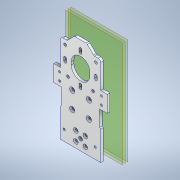
# Autodesk Inventor part: Printhead Base Plate REVI
Saved by Autodesk Inventor 2020 (Build 240168000, 168)
## iProperties
Created: 2023-06-15
Part Number: Printhead Base Plate REVI
Material: Aluminum 6061
Document SubType Name: Sheet Metal
Designer: Ishaan
Density: 2.7 g/cm^3
Appearance: Aluminum - Flat
Sheet Metal Rule: SendCutSend_1-8in_Alu
Author: Ishaan
Autodesk Inventor part; units mm, degrees
ref_plane "YZ Plane" through (0, 0, 0) normal (1, 0, 0) x (0, 1, 0)
ref_plane "XZ Plane" through (0, 0, 0) normal (0, 1, 0) x (-1, 0, 0)
ref_plane "XY Plane" through (0, 0, 0) normal (0, 0, 1) x (1, 0, 0)
sketch "Sketch1" plane through (0, 0, 0) normal (0, 0, 1) x (1, 0, 0)
  line L0 (31, -57.5) -> (-31, -57.5)
  line L1 (-31, -57.5) -> (-31, 57.5)
  line L2 (-31, 57.5) -> (31, 57.5)
  line L3 (31, 57.5) -> (31, -57.5)
  line L4 (31, -57.5) -> (-31, 57.5) construction
  line L5 (-31, -57.5) -> (31, 57.5) construction
  line L6 (-93.6831, -20.5) -> (93.6831, -20.5) construction
  line L7 (93.6831, -20.5) -> (93.6831, 1.5) construction
  line L8 (93.6831, 1.5) -> (-93.6831, 1.5) construction
  line L9 (-93.6831, 1.5) -> (-93.6831, -20.5) construction
  line L10 (-93.6831, -20.5) -> (93.6831, 1.5) construction
  line L11 (93.6831, -20.5) -> (-93.6831, 1.5) construction
  line L12 (22.7, -23) -> (-22.7, -23)
  line L13 (-22.7, -23) -> (-22.7, 4)
  line L14 (-22.7, 4) -> (22.7, 4)
  line L15 (22.7, 4) -> (22.7, -23)
  line L16 (22.7, -23) -> (-22.7, 4) construction
  line L17 (-22.7, -23) -> (22.7, 4) construction
  line L18 (-19.5, -44.75) -> (17.5, -44.75)
  circle A0 centre (0, -44.75) radius 8 construction
  line L19 (5.6569, -39.0931) -> (-5.6569, -39.0931) construction
  line L20 (-5.6569, -39.0931) -> (-5.6569, -50.4069) construction
  line L21 (-5.6569, -50.4069) -> (5.6569, -50.4069) construction
  line L22 (5.6569, -50.4069) -> (5.6569, -39.0931) construction
  line L23 (5.6569, -39.0931) -> (-5.6569, -50.4069) construction
  line L24 (-5.6569, -39.0931) -> (5.6569, -50.4069) construction
  line L25 (10, 0.5) -> (-10, 0.5)
  line L26 (-10, 0.5) -> (-10, -19.5)
  line L27 (-10, -19.5) -> (10, -19.5)
  line L28 (10, -19.5) -> (10, 0.5)
  line L29 (10, 0.5) -> (-10, -19.5) construction
  line L30 (-10, 0.5) -> (10, -19.5) construction
  point P0 (0, 0)
  point P1 (0, -9.5)
  point P2 (0, 0)
  point P3 (0, -9.5)
  point P4 (0, 0)
  dimension "d25" = 16
  dimension "d0" = 62
  dimension "d1" = 22
  dimension "d2" = 27
  dimension "d3" = 45.4
  dimension "d5" = 115
  dimension "d8" = 37
  dimension "d9" = 19.5
  dimension "d10" = 12.75
  dimension "d47" = 48
  dimension "d75" = 20
  dimension "d76" = 20
  constraints: 62 end point, 13 midpoint, 10 parallel, 7 coincident, 6 horizontal, 6 perpendicular, 2 vertical alignment, 1 point on line, 3 other
  measures "d0" distance of L1.end L2.end
  measures "d1" distance between parallel lines of L6 L8
  measures "d2" distance of L14.end L12.start
  measures "d3" distance of L13.end L14.end
  measures "d5" distance of L2.end L0.start
  measures "d8" distance of L18.start L18.end
  measures "d9" distance of point (0, -44.75) L18.start
  measures "d10" distance between parallel lines of L0 L18
  measures "d47" distance from line of L0 point (0, -9.5)
  measures "d75" distance of L27.end L26.end
  measures "d76" distance of L26.end L25.end
extrude "Extrusion1" add sketch "Sketch1" against normal blind 3.175 contours L0 L1 L2 L3 | L12 L13 L14 L15 | L28 L27 L26 L25
hole "Hole1" at (-19.5, -44.75, 0) at (17.5, -44.75, 0) direction (0, 0, -1) diameter 2.459 end through all thread size "M3x0.5" class "6H" standard "ANSI Metric M Profile"
hole "Hole2" at (0, -44.75, 0) direction (0, 0, -1) diameter 4.5 end through all
hole "Hole3" at (-5.6569, -50.4069, 0) at (5.6569, -50.4069, 0) at (-5.6569, -39.0931, 0) at (5.6569, -39.0931, 0) direction (0, 0, -1) diameter 2.9 end through all countersink diameter 5.5 countersink angle 90 clearance for "Flat Head Machine Screw" size "M2.5" standard "Ansi Metric M Profile"
sketch "Sketch2" plane through (0, 0, 0) normal (0, 0, 1) x (1, 0, 0)
  line L0 (21.9203, 28.8) -> (0, 6.8797) construction
  line L1 (0, 6.8797) -> (-21.9203, 28.8) construction
  line L2 (-21.9203, 28.8) -> (0, 50.7203) construction
  line L3 (0, 50.7203) -> (21.9203, 28.8) construction
  line L4 (21.9203, 28.8) -> (-21.9203, 28.8) construction
  line L5 (0, 6.8797) -> (0, 50.7203) construction
  line L6 (0, 28.8) -> (0, 31.8) construction
  line L7 (11.25, 28.8) -> (11.25, 31.8)
  line L8 (-11.25, 31.8) -> (-11.25, 28.8)
  arc A0 (-11.25, 28.8) -> (11.25, 28.8) centre (0, 28.8) ccw
  arc A1 (11.25, 31.8) -> (-11.25, 31.8) centre (0, 31.8) ccw
  line L9 (-21.9203, 28.8) -> (-21.9203, 31.8) construction
  line L10 (-20.2203, 28.8) -> (-20.2203, 31.8)
  line L11 (-23.6203, 31.8) -> (-23.6203, 28.8)
  arc A2 (-23.6203, 28.8) -> (-20.2203, 28.8) centre (-21.9203, 28.8) ccw
  arc A3 (-20.2203, 31.8) -> (-23.6203, 31.8) centre (-21.9203, 31.8) ccw
  line L12 (0, 6.8797) -> (0, 9.8797) construction
  line L13 (1.7, 6.8797) -> (1.7, 9.8797)
  line L14 (-1.7, 9.8797) -> (-1.7, 6.8797)
  arc A4 (-1.7, 6.8797) -> (1.7, 6.8797) centre (0, 6.8797) ccw
  arc A5 (1.7, 9.8797) -> (-1.7, 9.8797) centre (0, 9.8797) ccw
  line L15 (0, 50.7203) -> (0, 53.7203) construction
  line L16 (-1.7, 50.7203) -> (-1.7, 53.7203)
  line L17 (1.7, 53.7203) -> (1.7, 50.7203)
  arc A6 (-1.7, 50.7203) -> (1.7, 50.7203) centre (0, 50.7203) ccw
  arc A7 (1.7, 53.7203) -> (-1.7, 53.7203) centre (0, 53.7203) ccw
  circle A8 centre (-20, 13.3) radius 6.5 construction
  circle A9 centre (0, 6.8797) radius 3.5 construction
  circle A10 centre (20, 13.3) radius 6.5 construction
  line L18 (-20, 13.3) -> (20, 13.3) construction
  circle A11 centre (0, 30.3) radius 6.11 construction
  circle A12 centre (0, 30.3) radius 6.74 construction
  line L19 (-37.8272, 6.8) -> (-20, 6.8) construction
  line L20 (-13.8669, 11.147) -> (-6.3595, 32.5325) construction
  line L21 (6.3595, 32.5325) -> (13.8669, 11.147) construction
  line L22 (20, 6.8) -> (34.7774, 6.8) construction
  line L23 (21.9203, 28.8) -> (21.9203, 31.8) construction
  line L24 (23.6203, 28.8) -> (23.6203, 31.8)
  line L25 (20.2203, 31.8) -> (20.2203, 28.8)
  arc A13 (20.2203, 28.8) -> (23.6203, 28.8) centre (21.9203, 28.8) ccw
  arc A14 (23.6203, 31.8) -> (20.2203, 31.8) centre (21.9203, 31.8) ccw
  line L26 (29.6985, 28.8) -> (0, -0.8985) construction
  line L27 (0, -0.8985) -> (-29.6985, 28.8) construction
  line L28 (-29.6985, 28.8) -> (0, 58.4985) construction
  line L29 (0, 58.4985) -> (29.6985, 28.8) construction
  line L30 (29.6985, 28.8) -> (-29.6985, 28.8) construction
  line L31 (0, -0.8985) -> (0, 58.4985) construction
  circle A15 centre (-20, 13.3) radius 4 construction
  line L32 (93.6831, 1.5) -> (-93.6831, 1.5) construction
  point P0 (0, 0)
  point P1 (0, 28.8)
  point P2 (-21.9203, 30.3)
  point P3 (0, 8.3797)
  point P4 (0, 52.2203)
  point P5 (0, 13.3)
  point P6 (21.9203, 30.3)
  point P7 (0, -9.5)
  dimension "d33" = 31
  dimension "d34" = 31
  dimension "d35" = 22.5
  dimension "d36" = 1.7
  dimension "d37" = 3
  dimension "d38" = 13
  dimension "d39" = 7
  dimension "d40" = 12.22
  dimension "d41" = 0.63
  dimension "d42" = 42
  dimension "d43" = 8
  dimension "d45" = 40
  dimension "d52" = 17
  dimension "d86" = 5.3
  constraints: 74 end point, 26 point on circle, 26 tangent, 16 centre point, 11 midpoint, 9 parallel, 7 vertical, 5 equal length, 4 equal radius, 3 coincident, 2 perpendicular, 2 point on line, 2 vertical alignment, 1 horizontal
  measures "d33" distance of L1.end L2.end
  measures "d34" distance of L0.end L1.end
  measures "d35" diameter of A1
  measures "d36" radius of A3
  measures "d37" distance of L8.start L8.end
  measures "d38" diameter of A8
  measures "d39" diameter of A9
  measures "d40" diameter of A11
  measures "d41" radial gap between concentric circles of A11 A12
  measures "d42" distance of L27.end L28.end
  measures "d43" diameter of A15
  measures "d45" distance of L18.start L18.end
  measures "d52" distance from line of point (0, 30.3) L18
  measures "d86" distance between parallel lines of L19 L32
extrude "Extrusion2" [suppressed]
sketch "Sketch3" plane through (0, 0, 0) normal (0, 0, 1) x (1, 0, 0)
  line L0 (0, 50.8902) -> (24.8902, 26) construction
  line L1 (24.8902, 26) -> (0, 1.1098) construction
  line L2 (0, 1.1098) -> (-24.8902, 26) construction
  line L3 (-24.8902, 26) -> (0, 50.8902) construction
  line L4 (0, 50.8902) -> (0, 1.1098) construction
  line L5 (24.8902, 26) -> (-24.8902, 26) construction
  line L6 (0, 7.6152) -> (18.3848, 26) construction
  line L7 (18.3848, 26) -> (0, 44.3848) construction
  line L8 (0, 44.3848) -> (-18.3848, 26) construction
  line L9 (-18.3848, 26) -> (0, 7.6152) construction
  line L10 (0, 7.6152) -> (0, 44.3848) construction
  line L11 (18.3848, 26) -> (-18.3848, 26) construction
  line L12 (-18.3848, 26) -> (-18.3848, 29.5) construction
  line L13 (-16.7848, 26) -> (-16.7848, 29.5)
  line L14 (-19.9848, 29.5) -> (-19.9848, 26)
  arc A0 (-19.9848, 26) -> (-16.7848, 26) centre (-18.3848, 26) ccw
  arc A1 (-16.7848, 29.5) -> (-19.9848, 29.5) centre (-18.3848, 29.5) ccw
  line L15 (0, 44.3848) -> (0, 47.8848) construction
  line L16 (-1.6, 44.3848) -> (-1.6, 47.8848)
  line L17 (1.6, 47.8848) -> (1.6, 44.3848)
  arc A2 (-1.6, 44.3848) -> (1.6, 44.3848) centre (0, 44.3848) ccw
  arc A3 (1.6, 47.8848) -> (-1.6, 47.8848) centre (0, 47.8848) ccw
  line L18 (18.3848, 26) -> (18.3848, 29.5) construction
  line L19 (16.7848, 26) -> (16.7848, 29.5)
  line L20 (19.9848, 29.5) -> (19.9848, 26)
  arc A4 (16.7848, 26) -> (19.9848, 26) centre (18.3848, 26) ccw
  arc A5 (19.9848, 29.5) -> (16.7848, 29.5) centre (18.3848, 29.5) ccw
  line L21 (0, 7.6152) -> (0, 11.1152) construction
  line L22 (1.6, 7.6152) -> (1.6, 11.1152)
  line L23 (-1.6, 11.1152) -> (-1.6, 7.6152)
  arc A6 (-1.6, 7.6152) -> (1.6, 7.6152) centre (0, 7.6152) ccw
  arc A7 (1.6, 11.1152) -> (-1.6, 11.1152) centre (0, 11.1152) ccw
  line L24 (0, 26) -> (0, 29.5) construction
  line L25 (11.125, 26) -> (11.125, 29.5)
  line L26 (-11.125, 29.5) -> (-11.125, 26)
  arc A8 (-11.125, 26) -> (11.125, 26) centre (0, 26) ccw
  arc A9 (11.125, 29.5) -> (-11.125, 29.5) centre (0, 29.5) ccw
  circle A10 centre (0, 7.6152) radius 3.5 construction
  circle A11 centre (-15, 12) radius 6.5 construction
  circle A12 centre (15, 12) radius 6.5 construction
  line L27 (-15, 12) -> (15, 12) construction
  line L28 (93.6831, 1.5) -> (-93.6831, 1.5) construction
  circle A13 centre (0, 26) radius 6.11 construction
  circle A14 centre (0, 26) radius 6.74 construction
  line L29 (-8.5456, 11.2317) -> (-6.6927, 26.7967) construction
  line L30 (6.6927, 26.7967) -> (8.5456, 11.2317) construction
  line L31 (15, 5.5) -> (52.2336, 5.5) construction
  line L32 (-15, 5.5) -> (-44.4503, 5.5) construction
  circle A15 centre (-15, 12) radius 2 construction
  point P0 (0, 0)
  point P1 (-18.3848, 27.75)
  point P2 (0, 46.1348)
  point P3 (18.3848, 27.75)
  point P4 (0, 9.3652)
  point P5 (0, 27.75)
  point P6 (0, 12)
  dimension "d92" = 2.9
  dimension "d53" = 35.2
  dimension "d54" = 26
  dimension "d55" = 22.25
  dimension "d56" = 3.5
  dimension "d57" = 1.6
  dimension "d58" = 7
  dimension "d59" = 13
  dimension "d60" = 4
  dimension "d61" = 30
  dimension "d62" = 12.22
  dimension "d63" = 0.63
  dimension "d64" = 14
  dimension "d65" = 4
  constraints: 74 end point, 26 point on circle, 25 tangent, 16 centre point, 11 midpoint, 9 parallel, 6 equal length, 5 coincident, 4 equal radius, 4 perpendicular, 3 horizontal, 3 point on line, 2 vertical, 2 vertical alignment
  measures "d53" distance of L0.end L1.end
  measures "d54" distance of L7.end L8.end
  measures "d55" diameter of A9
  measures "d56" distance of L26.start L26.end
  measures "d57" radius of A1
  measures "d58" diameter of A10
  measures "d59" diameter of A11
  measures "d60" distance edge to line of A11 L28
  measures "d61" distance of L27.start L27.end
  measures "d62" diameter of A13
  measures "d63" radial gap between concentric circles of A13 A14
  measures "d64" distance between parallel lines of L5 L27
  measures "d65" diameter of A15
extrude "Extrusion3" cut sketch "Sketch3" against normal through all
hole "Hole4" at (-15, 12, 0) at (15, 12, 0) direction (0, 0, -1) diameter 3.242 end through all thread size "M4x0.7" class "6H" standard "ANSI Metric M Profile"
hole "Hole5" at (-10, -19.5, 0) at (-10, 0.5, 0) at (10, 0.5, 0) at (10, -19.5, 0) direction (0, 0, -1) diameter 3.2 end through all countersink diameter 6.3 countersink angle 90 clearance for "Flat Head Machine Screw" size "M3" standard "Ansi Metric M Profile"
ref_plane "Work Plane1" through (0, 0, -16.175) normal (0, 0, -1) x (-1, 0, 0)
ref_plane "Work Plane3" through (0, 0, -19.35) normal (0, 0, -1) x (-1, 0, 0)
ref_plane "Work Plane2" through (0, 0, -22.525) normal (0, 0, -1) x (-1, 0, 0)
sketch "Sketch4" plane through (0, 0, 0) normal (0, 0, 1) x (1, 0, 0)
  line L0 (-32, -2.65) -> (-22, -2.65)
  line L1 (-22, -2.65) -> (-22, 17.15)
  line L2 (-22, 17.15) -> (-32, 17.15)
  line L3 (-32, 17.15) -> (-32, -2.65)
  line L4 (-32, -2.65) -> (-22, 17.15) construction
  line L5 (-22, -2.65) -> (-32, 17.15) construction
  line L6 (-25, 12) -> (-25, 2.5) construction
  line L7 (-33.3, 34.9336) -> (-33.3, 2.4545) construction
  line L8 (-34.9, 35.6059) -> (-34.9, 1.9795) construction
  line L9 (-27.3543, -4.45) -> (-52.5717, -4.45) construction
  line L10 (93.6831, -15.5) -> (-93.6831, -15.5) construction
  line L11 (-93.6831, -15.5) -> (-93.6831, -3.5) construction
  line L12 (-93.6831, -3.5) -> (93.6831, -3.5) construction
  line L13 (93.6831, -3.5) -> (93.6831, -15.5) construction
  line L14 (93.6831, -15.5) -> (-93.6831, -3.5) construction
  line L15 (-93.6831, -15.5) -> (93.6831, -3.5) construction
  line L16 (-93.6831, 1.5) -> (-93.6831, -20.5) construction
  circle A0 centre (-25, 2.5) radius 1.7 construction
  circle A1 centre (-15, 12) radius 1.621 construction
  line L17 (-31, 57.5) -> (-31, -57.5) construction
  point P0 (0, 0)
  point P1 (-27, 7.25)
  point P2 (-25, 7.25)
  point P3 (-27, 7.25)
  point P4 (0, -9.5)
  point P5 (-27, 7.25)
  dimension "d87" = 10
  dimension "d88" = 19.8
  dimension "d89" = 9.5
  dimension "d90" = 7
  dimension "d91" = 1.3
  dimension "d92" = 2.9
  dimension "d93" = 1.8
  dimension "d94" = 12
  dimension "d95" = 3.4
  dimension "d103" = 16.75
  dimension "d104" = 1
  constraints: 32 end point, 7 midpoint, 4 parallel, 3 coincident, 3 horizontal, 3 vertical, 2 horizontal alignment, 2 perpendicular, 1 centre point, 1 point on line
  measures "d87" distance of L2.end L1.end
  measures "d88" distance of L1.end L0.end
  measures "d89" distance of L6.start L6.end
  measures "d90" distance between parallel lines of L3 L6
  measures "d91" distance between parallel lines of L3 L7
  measures "d92" distance between parallel lines of L8 L3
  measures "d93" distance between parallel lines of L9 L0
  measures "d94" distance of L10.end L11.end
  measures "d95" diameter of A0
  measures "d103" vertical distance of point (0, -9.5) point (-27, 7.25)
  measures "d104" distance between parallel lines of L17 L3
hole "Hole6" at (-25, 12, 0) at (-25, 2.5, 0) direction (0, 0, -1) diameter 2.459 end through all thread size "M3x0.5" class "6H" standard "ANSI Metric M Profile"
mirror "Mirror1" about plane through (0, 0, 0) normal (1, 0, 0) of "Hole6"
sketch "Sketch5" plane through (0, 0, 0) normal (0, 0, 1) x (1, 0, 0)
  line L0 (22.7, 4) -> (22.7, -23) projected
  line L1 (-22.7, -23) -> (-22.7, 4) projected
  line L2 (-31, -57.5) -> (31, -57.5) projected
  line L3 (-22.7, -2.65) -> (-32, -2.65)
  line L4 (-32, -2.65) -> (-32, 17.15)
  line L5 (-31, -57.5) -> (-31, 57.5) projected
  line L6 (-32, 17.15) -> (-24, 17.15)
  line L7 (-24, 17.15) -> (-24, 49)
  line L8 (-24, 49) -> (24, 49)
  line L9 (24, 49) -> (24, 17.15)
  line L10 (24, 17.15) -> (32, 17.15)
  line L11 (32, 17.15) -> (32, -2.65)
  line L12 (32, -2.65) -> (22.7, -2.65)
  line L13 (-32, -2.65) -> (-22, -2.65) projected
  line L14 (-32, 17.15) -> (-32, -2.65) projected
  line L15 (-32, 7.25) -> (32, 7.25) construction
  circle A0 centre (25, 12) radius 1.2295 projected
  circle A1 centre (25, 2.5) radius 1.2295 projected
  circle A2 centre (-25, 12) radius 1.2295 projected
  circle A3 centre (-25, 2.5) radius 1.2295 projected
  circle A4 centre (10, 0.5) radius 3.15 projected
  circle A5 centre (-10, -19.5) radius 3.15 projected
  circle A6 centre (-10, 0.5) radius 3.15 projected
  circle A7 centre (10, -19.5) radius 3.15 projected
  circle A8 centre (-15, 12) radius 1.621 projected
  circle A9 centre (15, 12) radius 1.621 projected
  arc A10 (-1.6, 44.3848) -> (1.6, 44.3848) centre (0, 44.3848) ccw projected
  line L16 (-1.6, 44.3848) -> (-1.6, 47.8848) projected
  arc A11 (1.6, 47.8848) -> (-1.6, 47.8848) centre (0, 47.8848) ccw projected
  line L17 (1.6, 47.8848) -> (1.6, 44.3848) projected
  line L18 (19.9848, 29.5) -> (19.9848, 26) projected
  arc A12 (16.7848, 26) -> (19.9848, 26) centre (18.3848, 26) ccw projected
  line L19 (16.7848, 26) -> (16.7848, 29.5) projected
  arc A13 (19.9848, 29.5) -> (16.7848, 29.5) centre (18.3848, 29.5) ccw projected
  line L20 (-16.7848, 29.5) -> (-16.7848, 26) projected
  arc A14 (-19.9848, 26) -> (-16.7848, 26) centre (-18.3848, 26) ccw projected
  line L21 (-19.9848, 26) -> (-19.9848, 29.5) projected
  arc A15 (-16.7848, 29.5) -> (-19.9848, 29.5) centre (-18.3848, 29.5) ccw projected
  arc A16 (1.6, 11.1152) -> (-1.6, 11.1152) centre (0, 11.1152) ccw projected
  line L22 (1.6, 11.1152) -> (1.6, 7.6152) projected
  arc A17 (-1.6, 7.6152) -> (1.6, 7.6152) centre (0, 7.6152) ccw projected
  line L23 (-1.6, 7.6152) -> (-1.6, 11.1152) projected
  arc A18 (11.125, 29.5) -> (-11.125, 29.5) centre (0, 29.5) ccw projected
  line L24 (11.125, 29.5) -> (11.125, 26) projected
  arc A19 (-11.125, 26) -> (11.125, 26) centre (0, 26) ccw projected
  line L25 (-11.125, 26) -> (-11.125, 29.5) projected
  circle A20 centre (-5.6569, -39.0931) radius 2.75 projected
  circle A21 centre (-5.6569, -50.4069) radius 2.75 projected
  circle A22 centre (5.6569, -50.4069) radius 2.75 projected
  circle A23 centre (5.6569, -39.0931) radius 2.75 projected
  circle A24 centre (0, -44.75) radius 2.25 projected
  circle A25 centre (-19.5, -44.75) radius 1.2295 projected
  circle A26 centre (17.5, -44.75) radius 1.2295 projected
  line L26 (31, 57.5) -> (-31, 57.5) projected
  line L27 (-31, 57.5) -> (-31, -57.5) projected
  line L28 (-31, -57.5) -> (31, -57.5) projected
  line L29 (31, -57.5) -> (31, 57.5) projected
  line L30 (16, 49) -> (7.5, 57.5)
  line L31 (-16, 49) -> (-7.5, 57.5)
  line L32 (-7.5, 57.5) -> (7.5, 57.5)
  line L33 (-31, 57.5) -> (31, 57.5) projected
  line L34 (24, -57.5) -> (-24, -57.5)
  line L35 (-24, -57.5) -> (-24, -23)
  line L36 (-24, -23) -> (24, -23)
  line L37 (24, -23) -> (24, -57.5)
  line L38 (24, -57.5) -> (-24, -23) construction
  line L39 (-24, -57.5) -> (24, -23) construction
  line L40 (22.7, -23) -> (-22.7, -23) projected
  point P0 (0, 0)
  point P1 (-19.5, -57.5)
  point P2 (22.7, -19)
  point P3 (-22.7, -19)
  point P4 (0, 49)
  point P5 (0, 7.25)
  point P6 (31, 17.15)
  point P7 (-31, 17.15)
  point P8 (-31, -2.65)
  point P9 (31, -2.65)
  point P10 (0, 57.5)
  point P11 (0, -40.25)
  point P12 (0, -23)
  point P13 (0, -9.5)
  point P14 (22.7, -23)
  point P15 (-22.7, -23)
  dimension "d107" = 48
  dimension "d110" = 135
  dimension "d111" = 135
  dimension "d112" = 15
  dimension "d130" = 48
  dimension "d131" = 37
  constraints: 38 end point, 10 point on line, 8 midpoint, 8 perpendicular, 7 collinear, 4 vertical alignment, 3 parallel, 2 horizontal
  measures "d107" distance between parallel lines of L9 L7
  measures "d110" angle of L31 L8
  measures "d111" angle of L8 L30
  measures "d112" distance of L31.end L30.end
  measures "d130" distance of L35.end L36.end
  measures "d131" distance from line of L8 A8.centre
extrude "Extrusion4" cut sketch "Sketch5" against normal through all contours L12 L29 L2 L37 L36 L0 | L36 L35 L2 L5 L3 L1 | L10 L9 L8 L30 L26 L29 | L5 L26 L31 L8 L7 L6 | A24 | A25 | A26
extrude "Extrusion5" add sketch "Sketch5" against normal up to surface (3.175 mm away) contours L29 L10 L11 L12 | L3 L4 L6 L5
chamfer "Chamfer1" distance 1.3 angle 45 2 edges at (22.7, -23, -1.5875) (-22.7, -23, -1.5875)
fillet "Fillet1" radius 3 2 edges at (-24, 49, -1.5875) (24, 49, -1.5875)
fillet "Fillet2" radius 2 4 edges at (-16, 49, -1.5875) (-7.5, 57.5, -1.5875) (7.5, 57.5, -1.5875) (16, 49, -1.5875)
sketch "Sketch6" plane through (0, 0, -3.175) normal (0, 0, -1) x (-1, 0, 0)
  line L0 (11.125, 29.5) -> (11.125, 26) projected
  arc A0 (-11.125, 26) -> (11.125, 26) centre (0, 26) ccw projected
  line L1 (-11.125, 26) -> (-11.125, 29.5) projected
  arc A1 (11.125, 29.5) -> (-11.125, 29.5) centre (0, 29.5) ccw projected
  line L2 (1.6, 11.1152) -> (1.6, 7.6152) projected
  arc A2 (-1.6, 7.6152) -> (1.6, 7.6152) centre (0, 7.6152) ccw projected
  line L3 (-1.6, 7.6152) -> (-1.6, 11.1152) projected
  arc A3 (1.6, 11.1152) -> (-1.6, 11.1152) centre (0, 11.1152) ccw projected
  arc A4 (16.7848, 26) -> (19.9848, 26) centre (18.3848, 26) ccw projected
  line L4 (16.7848, 26) -> (16.7848, 29.5) projected
  arc A5 (19.9848, 29.5) -> (16.7848, 29.5) centre (18.3848, 29.5) ccw projected
  line L5 (19.9848, 29.5) -> (19.9848, 26) projected
  arc A6 (-19.9848, 26) -> (-16.7848, 26) centre (-18.3848, 26) ccw projected
  line L6 (-19.9848, 26) -> (-19.9848, 29.5) projected
  arc A7 (-16.7848, 29.5) -> (-19.9848, 29.5) centre (-18.3848, 29.5) ccw projected
  line L7 (-16.7848, 29.5) -> (-16.7848, 26) projected
  line L8 (-1.6, 44.3848) -> (-1.6, 47.8848) projected
  arc A8 (1.6, 47.8848) -> (-1.6, 47.8848) centre (0, 47.8848) ccw projected
  line L9 (1.6, 47.8848) -> (1.6, 44.3848) projected
  arc A9 (-1.6, 44.3848) -> (1.6, 44.3848) centre (0, 44.3848) ccw projected
  circle A10 centre (-15, 12) radius 1.621 projected
  circle A11 centre (15, 12) radius 1.621 projected
  circle A12 centre (-10, -19.5) radius 1.6 projected
  circle A13 centre (10, 0.5) radius 1.6 projected
  circle A14 centre (10, -19.5) radius 1.6 projected
  circle A15 centre (-10, 0.5) radius 1.6 projected
  circle A16 centre (25, 2.5) radius 1.2295 projected
  circle A17 centre (25, 12) radius 1.2295 projected
  circle A18 centre (-25, 2.5) radius 1.2295 projected
  circle A19 centre (-25, 12) radius 1.2295 projected
  arc A20 (-6.6716, 57.5) -> (-8.0858, 56.9142) centre (-6.6716, 55.5) ccw projected
  line L10 (-8.0858, 56.9142) -> (-15.4142, 49.5858) projected
  arc A21 (-16.8284, 49) -> (-15.4142, 49.5858) centre (-16.8284, 51) ccw projected
  line L11 (-16.8284, 49) -> (-21, 49) projected
  arc A22 (-21, 49) -> (-24, 46) centre (-21, 46) ccw projected
  line L12 (-24, 46) -> (-24, 17.15) projected
  line L13 (-32, 17.15) -> (-24, 17.15) projected
  line L14 (-32, -2.65) -> (-32, 17.15) projected
  line L15 (-32, -2.65) -> (-22.7, -2.65) projected
  line L16 (-22.7, -2.65) -> (-22.7, -21.7) projected
  line L17 (22.7, -21.7) -> (22.7, -2.65) projected
  line L18 (32, -2.65) -> (22.7, -2.65) projected
  line L19 (32, 17.15) -> (32, -2.65) projected
  line L20 (32, 17.15) -> (24, 17.15) projected
  line L21 (24, 17.15) -> (24, 46) projected
  arc A23 (24, 46) -> (21, 49) centre (21, 46) ccw projected
  line L22 (21, 49) -> (16.8284, 49) projected
  arc A24 (15.4142, 49.5858) -> (16.8284, 49) centre (16.8284, 51) ccw projected
  line L23 (15.4142, 49.5858) -> (8.0858, 56.9142) projected
  arc A25 (8.0858, 56.9142) -> (6.6716, 57.5) centre (6.6716, 55.5) ccw projected
  line L24 (6.6716, 57.5) -> (-6.6716, 57.5) projected
  line L25 (-18.3848, 43.3848) -> (18.3848, 43.3848) construction
  line L26 (-24, -23) -> (-24, -57.5) projected
  line L27 (-24, -57.5) -> (24, -57.5) projected
  line L28 (24, -57.5) -> (24, -23) projected
  line L29 (-24, -23) -> (-22.7, -21.7) projected
  line L30 (22.7, -21.7) -> (24, -23) projected
  point P0 (0, 0)
  dimension "d120" = 5.6152
  dimension "d121" = 5.6152
  constraints: 2 coincident, 2 end point, 2 vertical alignment, 1 horizontal
  measures "d120" distance from line of L21 L25.end
  measures "d121" distance from line of L22 L25.end
hole "Hole7" at (18.3848, 43.3848, -3.175) at (-18.3848, 43.3848, -3.175) direction (0, 0, 1) diameter 3.242 end through all thread size "M4x0.7" class "6H" standard "ANSI Metric M Profile"
body "Solid1"
